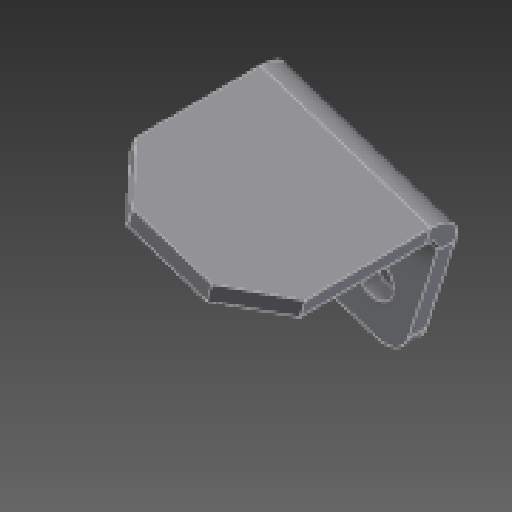
# Autodesk Inventor part: ChestBottomConnector
Saved by Autodesk Inventor 2025.2 (Build 292293000, 293)
## iProperties
Created: 2025-09-26
Part Number: ChestBottomConnector
Material: Generic
Document SubType Name: Sheet Metal
Designer: valer
Density: 1 g/cm^3
Sheet Metal Rule: Default
Appearance: Default
Author: valer
Autodesk Inventor part; units mm, degrees
ref_plane "YZ Plane" through (0, 0, 0) normal (1, 0, 0) x (0, 1, 0)
ref_plane "XZ Plane" through (0, 0, 0) normal (0, 1, 0) x (-1, 0, 0)
ref_plane "XY Plane" through (0, 0, 0) normal (0, 0, 1) x (1, 0, 0)
sketch "Sketch1" plane through (0, 0, 0) normal (0, 0, 1) x (1, 0, 0)
  circle A0 centre (29.4357, 133.8854) radius 3
  circle A1 centre (44.6474, 128.9251) radius 3
  line L0 (-87.8023, 180.5298) -> (92.7626, 121.6499) construction
  line L1 (29.4357, 133.8854) -> (44.6474, 128.9251) construction
  line L2 (25.2608, 143.6614) -> (53.7827, 134.3608)
  line L3 (53.7827, 134.3608) -> (48.8223, 119.1491)
  line L4 (25.2608, 143.6614) -> (20.3004, 128.4497)
  line L5 (20.3004, 128.4497) -> (48.8223, 119.1491)
  line L6 (37.0416, 131.4053) -> (39.5217, 139.0111) construction
  line L7 (25.2608, 143.6614) -> (26.1908, 146.5136)
  line L8 (26.1908, 146.5136) -> (54.7127, 137.213)
  line L9 (54.7127, 137.213) -> (53.7827, 134.3608)
  point P0 (0, 0)
  dimension "d0" = 30
  dimension "d20" = 3
  measures "d0" distance of L4.end L3.end
  measures "d20" distance between parallel lines of L8 L0
extrude "Plate1" add sketch "Sketch1" along normal blind 3.175
sketch "Sketch2" plane through (26.994, 148.9767, 5.7658) normal (0.3100206, 0.9507298, 0) x (-0.9507298, 0.3100206, 0)
  line L0 (-30, 0) -> (0, 0)
  line L1 (0, 0) -> (0, 29.2342)
  line L2 (0, 29.2342) -> (-30, 29.2342)
  line L3 (-30, 29.2342) -> (-30, 0)
  constraints: 6 end point, 1 horizontal, 1 perpendicular, 1 vertical
edge flange "FlangeFeature" height 35 angle 90 thickness 3.175 bend radius 2.5908 thickness toward (0.3100206, 0.9507298, 0) relief tear relief width 3.175 relief depth 1.5875 edges at (40.4518, 141.8633, 3.175) wall of the first edge with corners at (55.5159, 139.6761, 5.7658) (26.994, 148.9767, 5.7658) (26.994, 148.9767, 35) (55.5159, 139.6761, 35)
bend "Bend1"
corner "Corner1"
chamfer "ChamferFeature" distance 8 angle 45 2 edges at (27.4862, 150.486, 35) (56.0081, 141.1854, 35)
fillet "OutsideFilletsFeature" radius 4 2 edges at (20.3004, 128.4497, 1.5875) (48.8223, 119.1491, 1.5875)
sketch "MountHole" plane through (55.5159, 139.6761, 25.1089) normal (0.3100206, 0.9507298, 0) x (0.9507298, -0.3100206, 0)
  line L0 (-15, 19.3431) -> (-15, -9.8911) construction
  circle A0 centre (-15, 0.1089) radius 3.175
  line L1 (-30, 19.3431) -> (0, 19.3431) projected
  line L2 (-8, -9.8911) -> (-22, -9.8911) projected
  point P0 (-9.4782, 25.1089)
  dimension "d16" = 6.35
  dimension "d21" = 10
  constraints: 2 end point, 2 midpoint, 1 centre point, 1 point on line
  measures "d16" diameter of A0
  measures "d21" distance from line of L2 A0.centre
extrude "MountHoleFeature" cut sketch "MountHole" along normal through all both and the other way through all
equation "\"d18\" = Thickness"
equation "\"d1\" = Thickness"
equation "\"d2\" = BendReliefWidth"
equation "\"d3\" = BendReliefDepth"
equation "\"d4\" = MinimumRemnant"
equation "\"d5\" = TransitionRadius"
equation "\"d9\" = CornerReliefSize"
equation "\"d10\" = GapSize"
equation "\"d11\" = JacobiRadiusSize"
equation "\"BendRadius\" = Thickness"
equation "\"BendReliefWidth\" = Thickness"
equation "\"BendReliefDepth\" = 0.5 * Thickness"
equation "\"CornerReliefSize\" = 4 * Thickness"
equation "\"MinimumRemnant\" = 2 * Thickness"
equation "\"TransitionRadius\" = BendRadius"
equation "\"JacobiRadiusSize\" = BendRadius"
equation "\"GapSize\" = Thickness"
equation "\"Thickness\" = 3.175"
body "Solid1"
